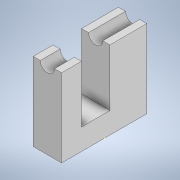
# Autodesk Inventor part: shaft_support
Saved by Autodesk Inventor 2021 (Build 250183000, 183)
## iProperties
Created: 2021-04-13
Part Number: shaft_support
Material: Generic
Document SubType Name: Modeling
Designer: Jawal
Density: 1 g/cm^3
Appearance: Default
Author: Jawal
Autodesk Inventor part; units mm, degrees
ref_plane "YZ Plane" through (0, 0, 0) normal (1, 0, 0) x (0, 1, 0)
ref_plane "XZ Plane" through (0, 0, 0) normal (0, 1, 0) x (-1, 0, 0)
ref_plane "XY Plane" through (0, 0, 0) normal (0, 0, 1) x (1, 0, 0)
sketch "Sketch1" plane through (0, 0, 0) normal (0, 1, 0) x (-1, 0, 0)
  line L0 (5, 15) -> (-5, 15)
  line L1 (-5, 15) -> (-5, -15)
  line L2 (-5, -15) -> (5, -15)
  line L3 (5, -15) -> (5, 15)
  point P0 (0, 0)
  dimension "d0" = 30
  dimension "d1" = 10
  dimension "d2" = 5
  dimension "d3" = 15
  constraints: 8 end point, 2 parallel, 1 horizontal, 1 perpendicular
  measures "d0" distance of L2.end L0.start
  measures "d1" distance of L1.end L2.end
  measures "d2" distance from line of L3 point (0, 0)
  measures "d3" distance from line of point (0, 0) L0
extrude "Extrusion1" add sketch "Sketch1" along normal blind 27.5
sketch "Sketch4" plane through (5, 0, 15) normal (1, 0, 0) x (0, 0, -1)
  point P0 (15, 0)
sketch "Sketch5" plane through (5, 0, 15) normal (1, 0, 0) x (0, 0, -1)
  line L0 (7, 27.5) -> (17, 27.5)
  line L1 (17, 27.5) -> (17, 7.5)
  line L2 (17, 7.5) -> (7, 7.5)
  line L3 (7, 7.5) -> (7, 27.5)
  line L4 (0, 0) -> (0, 27.5) projected
  line L5 (30, 0) -> (30, 27.5) projected
  point P0 (15, 0)
  dimension "d12" = 7
  dimension "d14" = 10
  dimension "d15" = 20
  constraints: 8 end point, 2 parallel, 1 horizontal, 1 perpendicular
  measures "d12" distance between parallel lines of L4 L3
  measures "d14" distance of L0.start L0.end
  measures "d15" distance of L0.end L1.end
extrude "Extrusion4" cut sketch "Sketch5" against normal through all
sketch "Sketch6" plane through (-5, 0, 15) normal (0, 0, 1) x (1, 0, 0)
  line L0 (10, 27.5) -> (0, 27.5) projected
  arc A0 (2.5, 27.5) -> (7.5, 27.5) centre (5, 27.5) ccw
  line L1 (2.5, 27.5) -> (7.5, 27.5)
  point P0 (5, 0)
  dimension "d18" = 5
  constraints: 2 end point, 2 point on circle, 2 point on line, 1 centre point, 1 collinear, 1 midpoint
  measures "d18" diameter of A0
extrude "Extrusion5" cut sketch "Sketch6" against normal through all
sketch "Sketch8" plane through (0, 0, 0) normal (0, -1, 0) x (1, 0, 0)
  circle A0 centre (0, -4) radius 1.5
  line L0 (5, -15) -> (-5, -15) projected
  line L1 (-5, 15) -> (5, 15) projected
  point P0 (0, 0)
  dimension "d24" = 3
  dimension "d28" = 19
  constraints: 1 centre point
  measures "d24" diameter of A0
  measures "d28" distance from line of L1 A0.centre
extrude "Extrusion6" add sketch "Sketch8" along normal blind 3
equation "\"d2\" = 0.5 * d1"
equation "\"d3\" = 0.5 * d0"
body "Solid1"
